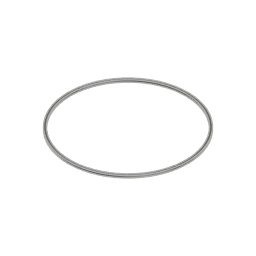
Partie Trappe Base Basse (Autodesk Fusion 360 archive; units mm, degrees)
design "Anneau Joint Torique Trappe"
Autodesk Fusion 360 part; units mm, degrees
sketch "Esquisse1" plane through (0, 0, 0) normal (0, 0, 1) x (1, 0, 0)
  circle A0 centre (0, 0) radius 27.9
  circle A1 centre (0, 0) radius 28.9
  dimension "d1" = 55.8
  dimension "d2" = 57.8
  constraint coincident A0.centre A1.centre
  measures "d1" diameter of A0
  measures "d2" diameter of A1
extrude "Extrusion1" add sketch "Esquisse1" along normal blind 1

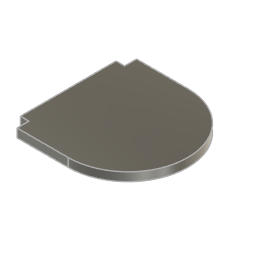
design "Couvercle"
Autodesk Fusion 360 part; units mm, degrees
sketch "Esquisse1" plane through (0, 0, 0) normal (0, 0, 1) x (1, 0, 0)
  line L0 (-17.5, 35) -> (17.5, 35)
  line L1 (17.5, 35) -> (17.5, -35)
  line L2 (17.5, -35) -> (-17.5, -35)
  line L3 (-17.5, -35) -> (-17.5, 35)
  line L4 (-17.5, 35) -> (17.5, -35) construction
  line L5 (17.5, 35) -> (-17.5, -35) construction
  arc A0 (17.5, -35) -> (17.5, 35) centre (17.5, 0) ccw
  line L6 (-17.5, 35) -> (-12.5, 35)
  line L7 (-12.5, 35) -> (-12.5, 28)
  line L8 (-12.5, 28) -> (-17.5, 28)
  line L9 (-17.5, 28) -> (-17.5, 35)
  line L10 (-17.5, -35) -> (-12.5, -35)
  line L11 (-12.5, -35) -> (-12.5, -28)
  line L12 (-12.5, -28) -> (-17.5, -28)
  line L13 (-17.5, -28) -> (-17.5, -35)
  dimension "d1" = 35
  dimension "d2" = 70
  dimension "d13" = 7
  dimension "d14" = 5
  dimension "d15" = 5
  dimension "d16" = 7
  constraint horizontal L0
  constraint perpendicular L0 L1
  constraint parallel L0 L2
  constraint parallel L1 L3
  constraint coincident L4 origin
  constraint coincident L5 origin
  constraint midpoint L1 A0.centre
  constraint horizontal L6
  constraint vertical L7
  constraint horizontal L8
  constraint vertical L9
  constraint horizontal L10
  constraint vertical L11
  constraint horizontal L12
  constraint vertical L13
  measures "d1" distance of L0.start L0.end
  measures "d2" distance of L0.end L1.end
  measures "d13" distance of L6.end L7.end
  measures "d14" distance of L7.end L8.end
  measures "d15" distance of L11.end L12.end
  measures "d16" distance of L10.end L11.end
extrude "Extrusion1" add sketch "Esquisse1" along normal blind 5 contours L0 L1 L2 L3 L7 L8 L11 L12 | L1 A0
